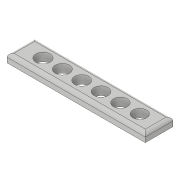
# Autodesk Inventor part: Bearing hole test
Saved by Autodesk Inventor 2019 (Build 230136000, 136)
## iProperties
Created: 2019-10-12
Part Number: Bearing hole test
Material: Generic
Document SubType Name: Modeling
Designer: ball
Density: 1 g/cm^3
Appearance: Default
Author: ball
Autodesk Inventor part; units mm, degrees
ref_plane "YZ Plane" through (0, 0, 0) normal (1, 0, 0) x (0, 1, 0)
ref_plane "XZ Plane" through (0, 0, 0) normal (0, 1, 0) x (-1, 0, 0)
ref_plane "XY Plane" through (0, 0, 0) normal (0, 0, 1) x (1, 0, 0)
sketch "Sketch1" plane through (0, 0, 0) normal (0, 1, 0) x (-1, 0, 0)
  line L0 (0, 0) -> (127, 0)
  line L1 (127, 0) -> (127, -25.4)
  line L2 (127, -25.4) -> (0, -25.4)
  line L3 (0, -25.4) -> (0, 0)
  dimension "d0" = 127
  dimension "d1" = 25.4
  constraints: 8 end point, 2 parallel, 1 horizontal, 1 perpendicular
  measures "d0" distance of L1.end L2.end
  measures "d1" distance of L0.end L1.end
extrude "Extrusion1" add sketch "Sketch1" along normal blind 7.62
sketch "Sketch2" plane through (0, 7.62, 0) normal (0, 1, 0) x (1, 0, 0)
  circle A0 centre (-17.78, 12.7) radius 6.2865
  circle A1 centre (-35.56, 12.7) radius 6.35
  circle A2 centre (-53.34, 12.7) radius 6.4135
  circle A3 centre (-71.12, 12.7) radius 6.477
  circle A4 centre (-88.9, 12.7) radius 6.5405
  circle A5 centre (-106.68, 12.7) radius 6.604
  line L0 (0, 0) -> (0, 25.4) projected
  dimension "d4" = 12.573
  dimension "d5" = 12.7
  dimension "d6" = 12.827
  dimension "d7" = 12.954
  dimension "d8" = 13.081
  dimension "d9" = 13.208
  dimension "d10" = 17.78
  dimension "d11" = 17.78
  dimension "d12" = 17.78
  dimension "d13" = 17.78
  dimension "d14" = 17.78
  dimension "d15" = 17.78
  constraints: 6 centre point
  measures "d4" diameter of A0
  measures "d5" diameter of A1
  measures "d6" diameter of A2
  measures "d7" diameter of A3
  measures "d8" diameter of A4
  measures "d9" diameter of A5
  measures "d10" distance from line of L0 A0.centre
  measures "d11" distance of A0.centre A1.centre
  measures "d12" distance of A1.centre A2.centre
  measures "d13" distance of A2.centre A3.centre
  measures "d14" distance of A3.centre A4.centre
  measures "d15" distance of A4.centre A5.centre
extrude "Extrusion2" cut sketch "Sketch2" against normal through all
fillet "Fillet1" radius 3.175 4 edges at (-63.5, 7.62, 0) (-63.5, 7.62, -25.4) (0, 7.62, -12.7) (-127, 7.62, -12.7)
body "Solid1"
